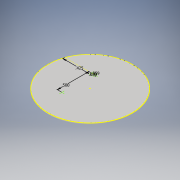
# Autodesk Inventor part: Replacemnet part(wall socket)
Saved by Autodesk Inventor 2018 (Build 220112000, 112)
## iProperties
Created: 2019-02-07
Part Number: Replacemnet part(wall socket)
Material: Generic
Document SubType Name: Modeling
Designer: This kid
Density: 1 g/cm^3
Appearance: Default
Author: This kid
Autodesk Inventor part; units mm, degrees
ref_plane "YZ Plane" through (0, 0, 0) normal (1, 0, 0) x (0, 1, 0)
ref_plane "XZ Plane" through (0, 0, 0) normal (0, 1, 0) x (-1, 0, 0)
ref_plane "XY Plane" through (0, 0, 0) normal (0, 0, 1) x (1, 0, 0)
sketch "Sketch1" plane through (0, 0, 0) normal (0, 1, 0) x (-1, 0, 0)
  circle A0 centre (0, 0) radius 16.9164
  dimension "d0" = 33.8328
  constraints: 1 centre point, 1 coincident
  measures "d0" diameter of A0
extrude "Extrusion1" add sketch "Sketch1" along normal blind 1
fillet "Fillet1" radius 1.016 1 edges at (16.9164, 0, 0)
sketch "Sketch2" plane through (0, 1, 0) normal (0, 1, 0) x (1, 0, 0)
  circle A0 centre (0, 0) radius 16.9164 projected
  line L0 (-4.3706, 5.7321) -> (-3.6206, 5.7321) construction
  line L1 (-4.3706, 5.7321) -> (-5.1206, 5.7321) construction
  line L2 (-5.1206, 5.7321) -> (-15.9156, 5.7321) construction
  point P0 (-4.3706, -6.9679)
  dimension "d8" = 12.7
  dimension "d10" = 1.5
  dimension "d14" = 0.75
  dimension "d15" = 0.75
  dimension "d16" = 10.795
  constraints: 6 end point, 2 horizontal, 2 other
  measures "d8" distance of point (-4.371, -6.968) L0.start
  measures "d10" distance of L0.end L1.end
  measures "d14" distance of L0.start L0.end
  measures "d15" distance of L0.start L1.end
  measures "d16" distance of L1.end L2.end
body "Solid1"
